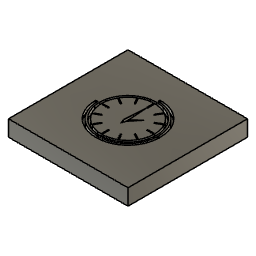
SignifierTemplate (Autodesk Fusion 360 design; units mm, degrees)
Autodesk Fusion 360 part; units mm, degrees
note: some values were not read from the file. Chosen so that the rebuilt part matches the saved one: which face or edge a step refers to. Set by a fixed rule: which sketch regions a step uses.
sketch "Surface Sketch" plane through (0, 0, 0) normal (0, 0, 1) x (1, 0, 0)
  line L0 (0, 0) -> (381, 0)
  line L1 (381, 0) -> (381, 381)
  line L2 (381, 381) -> (0, 381)
  line L3 (0, 381) -> (0, 0)
  dimension "d1" = 381
  dimension "d2" = 381
  constraint horizontal L0
  constraint vertical L1
  constraint horizontal L2
  constraint vertical L3
  constraint coincident L0.start L3.end
  measures "d1" distance of L0.start L0.end
  measures "d2" distance of L0.start L2.end
extrude "Extrude1" add sketch "Surface Sketch" along normal blind 50.8
sketch "stopwatch" plane through (87.7016, 43.5059, 50.8) normal (0, 0, 1) x (1, 0, 0)
  spline S0 degree 3 poles (174.4744, 107.0599) (174.8984, 106.1294) (174.1005, 104.9604) (173.0504, 104.9736) knots 0 0 0 0 1 1 1 1
  spline S1 degree 3 poles (103.2867, 197.6863) (103.0064, 202.307) (102.7185, 206.1281) (102.6469, 206.1777) knots 0 0 0 0 1 1 1 1
  spline S2 degree 3 poles (106.7663, 140.207) (106.5595, 143.9538) (105.6452, 159.1183) (104.4616, 178.4313) knots 0 0 0 0 1 1 1 1
  line L0 (163.7923, 109.8926) -> (163.7923, 109.8926)
  line L1 (106.9683, 136.5461) -> (106.7663, 140.207)
  spline S3 degree 3 poles (102.6469, 206.1777) (102.5753, 206.2273) (102.4217, 204.5866) (102.3055, 202.5316) knots 0 0 0 0 1 1 1 1
  spline S4 degree 3 poles (100.2513, 130.8086) (101.4191, 127.6456) (102.4361, 125.018) (102.5114, 124.9695) knots 0 0 0 0 1 1 1 1
  line L2 (104.8083, 130.7138) -> (104.8082, 130.7138)
  spline S5 degree 3 poles (102.3055, 202.5316) (102.1894, 200.4766) (101.2019, 184.7923) (100.1112, 167.6775) knots 0 0 0 0 1 1 1 1
  line L3 (104.8082, 130.7138) -> (106.9683, 136.5461)
  line L4 (98.128, 136.5596) -> (100.2513, 130.8086)
  spline S6 degree 3 poles (96.3492, 129.0079) (97.2033, 129.364) (97.9572, 129.7349) (98.0246, 129.8321) knots 0 0 0 0 1 1 1 1
  spline S7 degree 3 poles (98.0246, 129.8321) (98.1295, 129.9837) (97.5354, 131.7691) (96.6086, 134.087) knots 0 0 0 0 1 1 1 1
  line L5 (96.3492, 129.0079) -> (96.3492, 129.0079)
  spline S8 degree 3 poles (155.8184, 117.4758) (156.7041, 117.8126) (156.2597, 118.034) (166.2646, 112.2703) knots 0 0 0 0 1 1 1 1
  spline S9 degree 3 poles (104.4616, 178.4313) (104.0957, 184.4009) (103.567, 193.0656) (103.2867, 197.6863) knots 0 0 0 0 1 1 1 1
  spline S10 degree 3 poles (166.2646, 112.2703) (171.5278, 109.2382) (174.2768, 107.4936) (174.4744, 107.0599) knots 0 0 0 0 1 1 1 1
  spline S11 degree 3 poles (102.5114, 124.9695) (102.5867, 124.9211) (103.6202, 127.506) (104.8083, 130.7138) knots 0 0 0 0 1 1 1 1
  spline S12 degree 3 poles (173.0504, 104.9736) (172.5765, 104.9796) (168.9804, 106.8903) (163.7923, 109.8926) knots 0 0 0 0 1 1 1 1
  line L6 (100.1112, 167.6775) -> (98.128, 136.5596)
  spline S13 degree 3 poles (96.6086, 134.087) (96.3625, 134.7023) (96.3389, 134.7046) (96.0867, 134.1366) knots 0 0 0 0 1 1 1 1
  spline S14 degree 3 poles (96.0867, 134.1366) (95.2667, 132.2902) (94.1065, 128.1795) (94.4293, 128.2642) knots 0 0 0 0 1 1 1 1
  spline S15 degree 3 poles (94.4293, 128.2642) (94.6311, 128.3171) (95.495, 128.6517) (96.3492, 129.0079) knots 0 0 0 0 1 1 1 1
  spline S16 degree 3 poles (31.098, 148.6499) (42.3303, 148.725) (42.369, 148.7194) (42.369, 147.019) knots 0 0 0 0 1 1 1 1
  line L7 (108.6206, 147.2645) -> (108.8577, 144.0632)
  line L8 (119.4504, 157.0022) -> (108.6206, 147.2645)
  line L9 (20.6785, 145.8823) -> (20.6785, 145.8823)
  spline S17 degree 3 poles (131.7874, 167.7571) (132.6335, 168.8097) (130.953, 167.3447) (119.4504, 157.0022) knots 0 0 0 0 1 1 1 1
  line L10 (174.2854, 145.314) -> (164.2185, 145.314)
  spline S18 degree 3 poles (108.8577, 144.0632) (108.9881, 142.3024) (109.0715, 140.6301) (109.0431, 140.347) knots 0 0 0 0 1 1 1 1
  spline S19 degree 3 poles (20.5132, 148.0302) (20.8976, 148.5562) (21.3894, 148.585) (31.098, 148.6499) knots 0 0 0 0 1 1 1 1
  spline S20 degree 3 poles (31.2633, 145.323) (21.6193, 145.3141) (21.2256, 145.3351) (20.6785, 145.8823) knots 0 0 0 0 1 1 1 1
  spline S21 degree 3 poles (163.8634, 148.3646) (164.2113, 148.6342) (166.7319, 148.7018) (174.5011, 148.6499) knots 0 0 0 0 1 1 1 1
  spline S22 degree 3 poles (20.6785, 145.8823) (20.0095, 146.5513) (19.9545, 147.2657) (20.5132, 148.0302) knots 0 0 0 0 1 1 1 1
  spline S23 degree 3 poles (163.6246, 146.0691) (162.9797, 146.8889) (163.0692, 147.7492) (163.8634, 148.3646) knots 0 0 0 0 1 1 1 1
  spline S24 degree 3 poles (124.8346, 159.1294) (128.3812, 163.5294) (131.51, 167.4119) (131.7874, 167.7571) knots 0 0 0 0 1 1 1 1
  spline S25 degree 3 poles (174.5011, 148.6499) (184.2097, 148.585) (184.7015, 148.5562) (185.0859, 148.0302) knots 0 0 0 0 1 1 1 1
  spline S26 degree 3 poles (185.0859, 148.0302) (185.6446, 147.2657) (185.5897, 146.5513) (184.9207, 145.8823) knots 0 0 0 0 1 1 1 1
  spline S27 degree 3 poles (42.369, 147.019) (42.369, 145.3449) (42.2911, 145.333) (31.2633, 145.323) knots 0 0 0 0 1 1 1 1
  line L11 (164.2185, 145.314) -> (163.6246, 146.0691)
  spline S28 degree 3 poles (113.9143, 145.5391) (116.3739, 148.6137) (121.288, 154.7294) (124.8346, 159.1294) knots 0 0 0 0 1 1 1 1
  spline S29 degree 3 poles (184.9207, 145.8823) (184.3738, 145.3354) (183.9735, 145.314) (174.2854, 145.314) knots 0 0 0 0 1 1 1 1
  spline S30 degree 3 poles (73.327, 200.6132) (73.3508, 199.299) (71.9376, 198.5746) (70.9108, 199.3747) knots 0 0 0 0 1 1 1 1
  spline S31 degree 3 poles (174.4744, 186.978) (174.2768, 186.5443) (171.5278, 184.7997) (166.2646, 181.7676) knots 0 0 0 0 1 1 1 1
  spline S32 degree 3 poles (48.0993, 176.7631) (47.6305, 177.0097) (43.6861, 179.2622) (39.3341, 181.7687) knots 0 0 0 0 1 1 1 1
  line L12 (113.9143, 145.5391) -> (113.9143, 145.5391)
  spline S33 degree 3 poles (109.2168, 139.8906) (109.3409, 139.9223) (111.4547, 142.4645) (113.9143, 145.5391) knots 0 0 0 0 1 1 1 1
  spline S34 degree 3 poles (109.0431, 140.347) (109.0146, 140.0639) (109.0928, 139.8585) (109.2168, 139.8906) knots 0 0 0 0 1 1 1 1
  line L13 (48.0993, 176.7631) -> (48.0993, 176.7631)
  spline S35 degree 3 poles (32.5083, 189.0741) (33.3023, 189.0741) (49.8377, 179.7093) (50.4436, 178.9165) knots 0 0 0 0 1 1 1 1
  spline S36 degree 3 poles (166.2646, 181.7676) (158.7403, 177.433) (156.6403, 176.2644) (156.4479, 176.305) knots 0 0 0 0 1 1 1 1
  line L14 (155.7319, 176.5769) -> (155.7319, 176.5769)
  spline S37 degree 3 poles (50.4436, 178.9165) (51.5726, 177.4391) (49.8399, 175.8475) (48.0993, 176.7631) knots 0 0 0 0 1 1 1 1
  spline S38 degree 3 poles (173.0938, 189.0741) (174.1012, 189.0741) (174.8863, 187.882) (174.4744, 186.978) knots 0 0 0 0 1 1 1 1
  spline S39 degree 3 poles (39.3341, 181.7687) (34.07, 184.8006) (31.322, 186.5443) (31.1243, 186.978) knots 0 0 0 0 1 1 1 1
  spline S40 degree 3 poles (70.9108, 199.3747) (70.6601, 199.5701) (68.2615, 203.5324) (65.5804, 208.1798) knots 0 0 0 0 1 1 1 1
  spline S41 degree 3 poles (31.1243, 186.978) (30.7116, 187.8838) (31.4975, 189.0741) (32.5083, 189.0741) knots 0 0 0 0 1 1 1 1
  spline S42 degree 3 poles (155.7319, 176.5769) (154.9913, 176.8749) (154.6307, 178.0015) (155.0373, 178.7469) knots 0 0 0 0 1 1 1 1
  spline S43 degree 3 poles (156.4479, 176.305) (156.4011, 176.315) (156.0789, 176.4373) (155.7319, 176.5769) knots 0 0 0 0 1 1 1 1
  spline S44 degree 3 poles (65.5804, 208.1798) (60.3409, 217.2621) (60.1256, 217.8329) (61.6623, 218.5661) knots 0 0 0 0 1 1 1 1
  spline S45 degree 3 poles (155.0373, 178.7469) (155.4445, 179.4932) (172.1962, 189.0741) (173.0938, 189.0741) knots 0 0 0 0 1 1 1 1
  spline S46 degree 3 poles (61.6623, 218.5661) (62.2129, 218.8287) (62.5953, 218.8523) (62.9785, 218.6471) knots 0 0 0 0 1 1 1 1
  line L15 (70.9108, 199.3747) -> (70.9108, 199.3747)
  spline S47 degree 3 poles (62.9785, 218.6471) (63.7824, 218.2169) (73.3089, 201.6154) (73.327, 200.6132) knots 0 0 0 0 1 1 1 1
  spline S48 degree 3 poles (110.0453, 62.9086) (153.859, 66.8827) (187.1932, 103.2253) (187.1932, 147.019) knots 0 0 0 0 1 1 1 1
  spline S49 degree 3 poles (187.1932, 147.019) (187.1932, 193.6044) (149.3848, 231.4128) (102.7994, 231.4128) knots 0 0 0 0 1 1 1 1
  spline S50 degree 3 poles (32.5059, 104.9639) (32.035, 104.9639) (31.6045, 105.2217) (31.3004, 105.6859) knots 0 0 0 0 1 1 1 1
  line L16 (101.0741, 208.4539) -> (101.1553, 218.678)
  spline S51 degree 3 poles (103.7658, 207.857) (103.3484, 207.5287) (102.9135, 207.2601) (102.7994, 207.2601) knots 0 0 0 0 1 1 1 1
  spline S52 degree 3 poles (102.7994, 207.2601) (102.6852, 207.2601) (102.2504, 207.5287) (101.833, 207.857) knots 0 0 0 0 1 1 1 1
  line L17 (104.5246, 208.4539) -> (103.7658, 207.857)
  spline S53 degree 3 poles (137.107, 203.1398) (134.6355, 198.8884) (134.1113, 198.4355) (132.7848, 199.4055) knots 0 0 0 0 1 1 1 1
  spline S54 degree 3 poles (101.1553, 218.678) (101.2327, 228.4205) (101.2625, 228.9212) (101.7881, 229.3053) knots 0 0 0 0 1 1 1 1
  spline S55 degree 3 poles (155.0288, 115.3023) (154.6055, 116.0587) (155.0084, 117.1679) (155.8184, 117.4758) knots 0 0 0 0 1 1 1 1
  spline S56 degree 3 poles (39.3341, 112.2703) (49.339, 118.034) (48.8946, 117.8126) (49.7803, 117.4758) knots 0 0 0 0 1 1 1 1
  spline S57 degree 3 poles (142.6202, 218.6472) (143.4449, 219.0885) (144.6903, 218.3868) (144.8022, 217.4178) knots 0 0 0 0 1 1 1 1
  spline S58 degree 3 poles (49.7803, 117.4758) (50.5952, 117.166) (50.9869, 116.0726) (50.5631, 115.291) knots 0 0 0 0 1 1 1 1
  spline S59 degree 3 poles (50.5631, 115.291) (50.1587, 114.5451) (33.4057, 104.9639) (32.5059, 104.9639) knots 0 0 0 0 1 1 1 1
  spline S60 degree 3 poles (79.0723, 59.2429) (59.0508, 64.6897) (41.8591, 76.5174) (29.3, 93.4857) knots 0 0 0 0 1 1 1 1
  spline S61 degree 3 poles (29.3, 93.4857) (21.6334, 103.8439) (15.9676, 116.9549) (13.4724, 130.1117) knots 0 0 0 0 1 1 1 1
  spline S62 degree 3 poles (12.0286, 147.3031) (12.0462, 154.9866) (12.3954, 158.6792) (13.724, 165.2291) knots 0 0 0 0 1 1 1 1
  spline S63 degree 3 poles (13.724, 165.2291) (20.9417, 200.8105) (48.9937, 228.8474) (84.6408, 236.1075) knots 0 0 0 0 1 1 1 1
  spline S64 degree 3 poles (193.0513, 135.7948) (190.1656, 114.8463) (181.5528, 97.2922) (167.0395, 82.7788) knots 0 0 0 0 1 1 1 1
  spline S65 degree 3 poles (102.7994, 231.4128) (56.2311, 231.4128) (18.4055, 193.5873) (18.4055, 147.019) knots 0 0 0 0 1 1 1 1
  spline S66 degree 3 poles (132.7848, 199.4055) (132.4725, 199.6339) (132.2629, 200.1271) (132.2717, 200.6132) knots 0 0 0 0 1 1 1 1
  spline S67 degree 3 poles (102.7994, 237.7731) (112.5297, 237.7731) (118.6776, 236.9876) (126.9768, 234.6839) knots 0 0 0 0 1 1 1 1
  line L18 (110.0453, 62.9086) -> (110.0454, 62.9086)
  spline S68 degree 3 poles (144.8022, 217.4178) (144.8901, 216.656) (143.9461, 214.9046) (137.107, 203.1398) knots 0 0 0 0 1 1 1 1
  line L19 (31.3004, 105.6859) -> (31.3004, 105.6859)
  line L20 (132.7848, 199.4055) -> (132.7848, 199.4055)
  spline S69 degree 3 poles (13.4724, 130.1117) (12.281, 136.3943) (12.0111, 139.6077) (12.0286, 147.3031) knots 0 0 0 0 1 1 1 1
  spline S70 degree 3 poles (96.69, 56.253) (89.3994, 56.9514) (84.3382, 57.8104) (79.0723, 59.2429) knots 0 0 0 0 1 1 1 1
  spline S71 degree 3 poles (163.7923, 109.8926) (159.1265, 112.5926) (155.1829, 115.027) (155.0288, 115.3023) knots 0 0 0 0 1 1 1 1
  spline S72 degree 3 poles (103.8106, 229.3053) (104.3362, 228.9212) (104.3661, 228.4205) (104.4434, 218.678) knots 0 0 0 0 1 1 1 1
  line L21 (104.4434, 218.678) -> (104.5246, 208.4539)
  spline S73 degree 3 poles (126.9768, 234.6839) (148.836, 228.6163) (167.815, 214.4792) (179.8594, 195.2925) knots 0 0 0 0 1 1 1 1
  spline S74 degree 3 poles (179.8594, 195.2925) (186.8065, 184.2259) (191.1654, 171.9569) (193.0727, 158.101) knots 0 0 0 0 1 1 1 1
  spline S75 degree 3 poles (132.2717, 200.6132) (132.2898, 201.6154) (141.8163, 218.2169) (142.6202, 218.6472) knots 0 0 0 0 1 1 1 1
  line L22 (101.833, 207.857) -> (101.0741, 208.4539)
  spline S76 degree 3 poles (84.6408, 236.1075) (91.445, 237.4933) (94.4957, 237.7731) (102.7994, 237.7731) knots 0 0 0 0 1 1 1 1
  spline S77 degree 3 poles (193.0727, 158.101) (193.7676, 153.0526) (193.756, 140.9102) (193.0513, 135.7948) knots 0 0 0 0 1 1 1 1
  spline S78 degree 3 poles (167.0395, 82.7788) (152.5886, 68.328) (134.85, 59.5943) (114.266, 56.7955) knots 0 0 0 0 1 1 1 1
  line L23 (96.69, 56.253) -> (96.69, 56.253)
  spline S79 degree 3 poles (18.4055, 147.019) (18.4055, 105.5505) (48.5292, 70.2636) (89.5861, 63.6378) knots 0 0 0 0 1 1 1 1
  spline S80 degree 3 poles (114.266, 56.7955) (111.0918, 56.3639) (99.3238, 56.0007) (96.69, 56.253) knots 0 0 0 0 1 1 1 1
  line L24 (101.833, 207.857) -> (101.833, 207.857)
  spline S81 degree 3 poles (101.7881, 229.3053) (102.4877, 229.8165) (103.1111, 229.8165) (103.8106, 229.3053) knots 0 0 0 0 1 1 1 1
  spline S82 degree 3 poles (70.9108, 94.6632) (71.9373, 95.4631) (73.3504, 94.739) (73.3276, 93.4247) knots 0 0 0 0 1 1 1 1
  spline S83 degree 3 poles (101.7881, 64.7327) (101.2596, 65.1189) (101.2365, 65.5678) (101.2365, 75.4287) knots 0 0 0 0 1 1 1 1
  spline S84 degree 3 poles (65.5804, 85.8581) (68.2615, 90.5055) (70.6601, 94.4678) (70.9108, 94.6632) knots 0 0 0 0 1 1 1 1
  spline S85 degree 3 poles (142.3652, 75.6182) (141.3772, 76.4774) (132.2869, 92.5132) (132.2711, 93.4247) knots 0 0 0 0 1 1 1 1
  line L25 (102.0179, 86.3052) -> (102.7994, 86.8888)
  spline S86 degree 3 poles (61.5967, 75.4934) (60.1449, 76.2242) (60.3888, 76.8589) (65.5804, 85.8581) knots 0 0 0 0 1 1 1 1
  line L26 (101.7881, 64.7327) -> (101.7881, 64.7327)
  spline S87 degree 3 poles (103.8106, 64.7327) (103.5073, 64.511) (103.0522, 64.3295) (102.7994, 64.3295) knots 0 0 0 0 1 1 1 1
  spline S88 degree 3 poles (102.7994, 64.3295) (102.5465, 64.3295) (102.0915, 64.511) (101.7881, 64.7327) knots 0 0 0 0 1 1 1 1
  line L27 (102.7994, 86.8888) -> (103.5808, 86.3052)
  spline S89 degree 3 poles (31.3004, 105.6859) (30.9352, 106.2432) (30.895, 106.5567) (31.1243, 107.0599) knots 0 0 0 0 1 1 1 1
  spline S90 degree 3 poles (132.2711, 93.4247) (132.2484, 94.739) (133.6614, 95.4631) (134.6879, 94.6632) knots 0 0 0 0 1 1 1 1
  spline S91 degree 3 poles (73.3276, 93.4247) (73.3119, 92.518) (64.2245, 76.4803) (63.2417, 75.6247) knots 0 0 0 0 1 1 1 1
  spline S92 degree 3 poles (134.6879, 94.6632) (135.4644, 94.0581) (144.8545, 77.5244) (144.8545, 76.7621) knots 0 0 0 0 1 1 1 1
  line L28 (103.5808, 86.3052) -> (104.3622, 85.7215)
  line L29 (104.3622, 85.7215) -> (104.3622, 75.4287)
  spline S93 degree 3 poles (63.2417, 75.6247) (62.5649, 75.0356) (62.5142, 75.0316) (61.5967, 75.4934) knots 0 0 0 0 1 1 1 1
  spline S94 degree 3 poles (104.3622, 75.4287) (104.3622, 65.5678) (104.339, 65.1189) (103.8106, 64.7327) knots 0 0 0 0 1 1 1 1
  line L30 (61.5967, 75.4934) -> (61.5967, 75.4934)
  spline S95 degree 3 poles (144.8545, 76.7621) (144.8545, 75.5048) (143.3112, 74.7955) (142.3652, 75.6182) knots 0 0 0 0 1 1 1 1
  spline S96 degree 3 poles (31.1243, 107.0599) (31.3219, 107.4936) (34.0709, 109.2382) (39.3341, 112.2703) knots 0 0 0 0 1 1 1 1
  line L31 (101.2365, 85.7215) -> (102.0179, 86.3052)
  line L32 (142.3652, 75.6182) -> (142.3652, 75.6182)
  spline S97 degree 3 poles (89.5861, 63.6378) (95.6556, 62.6583) (104.0052, 62.3607) (110.0453, 62.9086) knots 0 0 0 0 1 1 1 1
  line L33 (101.2365, 75.4287) -> (101.2365, 85.7215)
extrude "Extrude2" cut sketch "stopwatch" against normal blind 12.7 contours S0 S8 S10 S12 S55 S71 | S1 S2 L1 S3 S4 S5 L3 L4 S9 S11 L6 | S16 S19 S20 S22 S27 | L7 L8 S17 S18 S24 S28 S33 S34 | L10 S21 S23 S25 S26 L11 S29 | S30 S40 S44 S46 S47 | S31 S36 S38 S42 S43 S45 | S32 S35 S37 S39 S41 | S50 S56 S58 S59 S89 S96 | L16 S51 S52 L17 S54 S72 L21 L22 S81 | S53 S57 S66 S68 S75 | S60 S61 S62 S63 S64 S67 S69 S70 S73 S74 S76 S77 S78 S80 | S82 S84 S86 S91 S93 | S83 L25 S87 S88 L27 L28 L29 S94 L31 L33 | S85 S90 S92 S95
sketch "Short Timer Sketch" plane through (0, 0, 50.8) normal (0, 0, 1) x (-1, 0, 0)
  line L0 (0, -381) -> (0, 0)
  line L1 (0, 0) -> (-381, 0)
  line L2 (-381, 0) -> (-381, -381)
  line L3 (-381, -381) -> (0, -381)
  spline S0 degree 3 poles (-280.7528, -179.3007) (-277.8672, -158.3522) (-269.2544, -140.7981) (-254.741, -126.2847) knots 0 0 0 0 1 1 1 1
  spline S1 degree 3 poles (-254.741, -126.2847) (-240.2902, -111.8339) (-222.5516, -103.1002) (-201.9676, -100.3014) knots 0 0 0 0 1 1 1 1
  spline S2 degree 3 poles (-201.9676, -100.3014) (-198.7933, -99.8699) (-187.0255, -99.5066) (-184.3916, -99.7589) knots 0 0 0 0 0.999998 0.999998 0.999998 0.999998
  spline S3 degree 3 poles (-184.3916, -99.7589) (-177.1009, -100.4573) (-172.0398, -101.3163) (-166.7739, -102.7488) knots 0 0 0 0 1 1 1 1
  spline S4 degree 3 poles (-166.7739, -102.7488) (-146.7523, -108.1956) (-129.5606, -120.0233) (-117.0015, -136.9916) knots 0 0 0 0 1 1 1 1
  spline S5 degree 3 poles (-117.0015, -136.9916) (-109.3349, -147.3498) (-103.6691, -160.4608) (-101.174, -173.6176) knots 0 0 0 0 1 1 1 1
  spline S6 degree 3 poles (-101.174, -173.6176) (-99.9825, -179.9002) (-99.7127, -183.1136) (-99.7302, -190.809) knots 0 0 0 0 1 1 1 1
  spline S7 degree 3 poles (-99.7302, -190.809) (-99.7478, -198.4925) (-100.097, -202.1851) (-101.4256, -208.735) knots 0 0 0 0 1 1 1 1
  spline S8 degree 3 poles (-101.4256, -208.735) (-108.6432, -244.3164) (-136.6953, -272.3533) (-172.3424, -279.6134) knots 0 0 0 0 1 1 1 1
  spline S9 degree 3 poles (-172.3424, -279.6134) (-179.1466, -280.9992) (-182.1973, -281.279) (-190.5009, -281.279) knots 0 0 0 0 1 1 1 1
  spline S10 degree 3 poles (-190.5009, -281.279) (-200.2312, -281.279) (-206.3792, -280.4935) (-214.6784, -278.1898) knots 0 0 0 0 1 1 1 1
  spline S11 degree 3 poles (-214.6784, -278.1898) (-236.5375, -272.1222) (-255.5166, -257.9851) (-267.561, -238.7984) knots 0 0 0 0 1 1 1 1
  spline S12 degree 3 poles (-267.561, -238.7984) (-274.5081, -227.7318) (-278.8669, -215.4628) (-280.7742, -201.6069) knots 0 0 0 0 1 1 1 1
  spline S13 degree 3 poles (-280.7742, -201.6069) (-281.4692, -196.5586) (-281.4575, -184.4161) (-280.7528, -179.3007) knots 0 0 0 0 1 1 1 1
  line L4 (0, -190.5) -> (-381, -190.5) construction
  line L5 (-190.5, 0) -> (-190.5, -381) construction
  line L6 (-190.5009, -286.359) -> (-190.5009, -292.709)
  line L7 (-286.3684, -190.5) -> (-292.7184, -190.5)
  line L8 (-190.5009, -292.709) -> (-193.0409, -292.709)
  line L9 (-190.5009, -286.359) -> (-193.0409, -286.359)
  line L10 (-292.7184, -190.5) -> (-292.7184, -193.04)
  line L11 (-286.3684, -190.5) -> (-286.3684, -193.04)
  arc A0 (-292.7184, -193.04) -> (-193.0409, -292.709) centre (-193.0409, -193.0315) ccw
  arc A1 (-286.3684, -193.04) -> (-193.0409, -286.359) centre (-193.0494, -193.04) ccw
  point P0 (-190.5009, -281.279)
  point P1 (-281.2884, -190.5)
  dimension "d7" = 6.35
  dimension "d8" = 6.35
  dimension "d9" = 2.54
  dimension "d10" = 2.54
  dimension "d11" = 2.54
  dimension "d12" = 2.54
  dimension "d13" = 5.08
  dimension "d14" = 5.08
  constraint midpoint L0 L4.start
  constraint midpoint L2 L4.end
  constraint midpoint L1 L5.start
  constraint midpoint L3 L5.end
  constraint coincident P0 S9.end
  constraint coincident L4 P1
  constraint coincident S13 P1
  constraint parallel L5 L6
  constraint coincident L4 L7.start
  constraint parallel L4 L7
  constraint perpendicular L5 L8
  constraint perpendicular L5 L9
  constraint perpendicular L4 L10
  constraint perpendicular L4 L11
  constraint vertical P0 L6.start
  constraint tangent L8 A0
  constraint tangent L11 A1
  measures "d7" distance of L6.start L6.end
  measures "d8" distance of L7.start L7.end
  measures "d9" distance of L6.end L8.end
  measures "d10" distance of L6.start L9.end
  measures "d11" distance of L7.end L10.end
  measures "d12" distance of L7.start L11.end
  measures "d13" distance of P1 L7.start
  measures "d14" distance of P0 L6.start
sketch "Long Timer Sketch" plane through (0, 0, 50.8) normal (0, 0, 1) x (-1, 0, 0)
  line L0 (0, -381) -> (0, 0)
  line L1 (0, 0) -> (-381, 0)
  line L2 (-381, 0) -> (-381, -381)
  line L3 (-381, -381) -> (0, -381)
  spline S0 degree 3 poles (-280.7528, -179.3007) (-277.8672, -158.3522) (-269.2544, -140.7981) (-254.741, -126.2847) knots 0 0 0 0 1 1 1 1
  spline S1 degree 3 poles (-254.741, -126.2847) (-240.2902, -111.8339) (-222.5516, -103.1002) (-201.9676, -100.3014) knots 0 0 0 0 1 1 1 1
  spline S2 degree 3 poles (-201.9676, -100.3014) (-198.7933, -99.8699) (-187.0255, -99.5066) (-184.3916, -99.7589) knots 0 0 0 0 0.999998 0.999998 0.999998 0.999998
  spline S3 degree 3 poles (-184.3916, -99.7589) (-177.1009, -100.4573) (-172.0398, -101.3163) (-166.7739, -102.7488) knots 0 0 0 0 1 1 1 1
  spline S4 degree 3 poles (-166.7739, -102.7488) (-146.7523, -108.1956) (-129.5606, -120.0233) (-117.0015, -136.9916) knots 0 0 0 0 1 1 1 1
  spline S5 degree 3 poles (-117.0015, -136.9916) (-109.3349, -147.3498) (-103.6691, -160.4608) (-101.174, -173.6176) knots 0 0 0 0 1 1 1 1
  spline S6 degree 3 poles (-101.174, -173.6176) (-99.9825, -179.9002) (-99.7127, -183.1136) (-99.7302, -190.809) knots 0 0 0 0 1 1 1 1
  spline S7 degree 3 poles (-99.7302, -190.809) (-99.7478, -198.4925) (-100.097, -202.1851) (-101.4256, -208.735) knots 0 0 0 0 1 1 1 1
  spline S8 degree 3 poles (-101.4256, -208.735) (-108.6432, -244.3164) (-136.6953, -272.3533) (-172.3424, -279.6134) knots 0 0 0 0 1 1 1 1
  spline S9 degree 3 poles (-172.3424, -279.6134) (-179.1466, -280.9992) (-182.1973, -281.279) (-190.5009, -281.279) knots 0 0 0 0 1 1 1 1
  spline S10 degree 3 poles (-190.5009, -281.279) (-200.2312, -281.279) (-206.3792, -280.4935) (-214.6784, -278.1898) knots 0 0 0 0 1 1 1 1
  spline S11 degree 3 poles (-214.6784, -278.1898) (-236.5375, -272.1222) (-255.5166, -257.9851) (-267.561, -238.7984) knots 0 0 0 0 1 1 1 1
  spline S12 degree 3 poles (-267.561, -238.7984) (-274.5081, -227.7318) (-278.8669, -215.4628) (-280.7742, -201.6069) knots 0 0 0 0 1 1 1 1
  spline S13 degree 3 poles (-280.7742, -201.6069) (-281.4692, -196.5586) (-281.4575, -184.4161) (-280.7528, -179.3007) knots 0 0 0 0 1 1 1 1
  line L4 (-190.5, -381) -> (-190.5, 0) construction
  line L5 (0, -190.5) -> (-381, -190.5) construction
  arc A0 (-286.3684, -193.04) -> (-193.0409, -286.359) centre (-193.0494, -193.04) ccw construction
  arc A1 (-292.7184, -193.04) -> (-193.0409, -292.709) centre (-193.0409, -193.0315) ccw construction
  line L6 (-190.5009, -286.359) -> (-193.0409, -286.359) construction
  line L7 (-190.5009, -286.359) -> (-190.5009, -292.709) construction
  line L8 (-190.5009, -292.709) -> (-193.0409, -292.709) construction
  line L9 (-286.3684, -190.5) -> (-292.7184, -190.5) construction
  line L10 (-292.7184, -190.5) -> (-292.7184, -193.04) construction
  line L11 (-286.3684, -190.5) -> (-286.3684, -193.04) construction
  line L12 (-190.5, -94.6303) -> (-190.5, -88.2803)
  line L13 (-190.5, -94.6303) -> (-193.04, -94.6303)
  line L14 (-190.5, -88.2803) -> (-193.04, -88.2803)
  line L15 (-286.3684, -190.5) -> (-286.3684, -187.96)
  line L16 (-292.7184, -190.5) -> (-292.7184, -187.96)
  arc A2 (-193.04, -94.6303) -> (-286.3684, -187.96) centre (-193.04, -187.9587) ccw
  arc A3 (-193.04, -88.2803) -> (-292.7184, -187.96) centre (-193.0387, -187.96) ccw
  line L17 (-190.5, -94.6303) -> (-187.96, -94.6303)
  line L18 (-190.5, -88.2803) -> (-187.96, -88.2803)
  line L19 (-94.6497, -190.5) -> (-88.2997, -190.5)
  line L20 (-88.2997, -190.5) -> (-88.2997, -187.96)
  line L21 (-94.6497, -190.5) -> (-94.6497, -187.96)
  arc A4 (-88.2997, -187.96) -> (-187.96, -88.2803) centre (-187.9793, -187.96) ccw
  arc A5 (-94.6497, -187.96) -> (-187.96, -94.6303) centre (-187.96, -187.9407) ccw
  line L22 (-286.3684, -190.5) -> (-286.3684, -193.04)
  line L23 (-292.7184, -190.5) -> (-292.7184, -193.04)
  line L24 (-190.5009, -286.359) -> (-190.5009, -292.709)
  line L25 (-190.5009, -292.709) -> (-193.0409, -292.709)
  line L26 (-190.5009, -286.359) -> (-193.0409, -286.359)
  arc A6 (-292.7184, -193.04) -> (-193.0409, -292.709) centre (-193.0409, -193.0315) ccw
  arc A7 (-286.3684, -193.04) -> (-193.0409, -286.359) centre (-193.0409, -193.0315) ccw
  point P0 (-190.5, -99.7103)
  point P1 (-99.7297, -190.5)
  dimension "d15" = 6.35
  dimension "d16" = 5.08
  dimension "d17" = 2.54
  dimension "d18" = 2.54
  dimension "d19" = 2.54
  dimension "d20" = 2.54
  dimension "d21" = 2.54
  dimension "d22" = 2.54
  dimension "d23" = 6.35
  dimension "d24" = 5.08
  dimension "d25" = 2.54
  dimension "d26" = 2.54
  constraint midpoint L3 L4.start
  constraint midpoint L1 L4.end
  constraint midpoint L0 L5.start
  constraint midpoint L2 L5.end
  constraint coincident L4 L12.start
  constraint parallel L4 L12
  constraint coincident S2 P0
  constraint coincident L4 P0
  constraint perpendicular L4 L13
  constraint perpendicular L4 L14
  constraint coincident L9.start L11.start
  constraint perpendicular L5 L15
  constraint coincident L9.end L10.start
  constraint perpendicular L5 L16
  constraint tangent L13 A2
  constraint tangent L16 A3
  constraint perpendicular L12 L17
  constraint perpendicular L12 L18
  constraint parallel L5 L19
  constraint coincident S6 P1
  constraint coincident L5 P1
  constraint horizontal L19.start P1
  constraint perpendicular L5 L20
  constraint perpendicular L19 L21
  constraint tangent L20 A4
  constraint tangent L17 A5
  constraint coincident A0.start L11.end
  constraint coincident A1.start L10.end
  constraint coincident L6.start L7.start
  constraint coincident L7.end L8.start
  constraint coincident A1.end L8.end
  constraint coincident A0.end L6.end
  constraint tangent L8 A6
  constraint tangent L26 A7
  measures "d15" distance of L12.start L12.end
  measures "d16" distance of L12.start P0
  measures "d17" distance of L12.start L13.end
  measures "d18" distance of L12.end L14.end
  measures "d19" distance of L9.start L15.end
  measures "d20" distance of L9.end L16.end
  measures "d21" distance of L12.start L17.end
  measures "d22" distance of L12.end L18.end
  measures "d23" distance of L19.start L19.end
  measures "d24" horizontal distance of L19.start P1
  measures "d25" distance of L19.end L20.end
  measures "d26" distance of L19.start L21.end
extrude "Extrude3" cut sketch "Short Timer Sketch" sketch "Long Timer Sketch" against normal blind 12.7 contours L6 L7 L8 L9 L10 L11 A0 A1 of sketch 2 contours L12 L13 L14 L15 L16 A2 A3 L22 L23 L24 L25 L26 A6 A7 | L12 L17 L18 L19 L20 L21 A4 A5
named bodies: "Surface"
